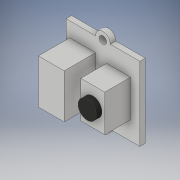
# Autodesk Inventor part: button
Saved by Autodesk Inventor 2019 (Build 230136000, 136)
## iProperties
Created: 2018-06-15
Part Number: button
Material: Generic
Document SubType Name: Modeling
Designer: daniel
Density: 1 g/cm^3
Appearance: Default
Author: daniel
Autodesk Inventor part; units mm, degrees
ref_plane "YZ Plane" through (0, 0, 0) normal (1, 0, 0) x (0, 1, 0)
ref_plane "XZ Plane" through (0, 0, 0) normal (0, 1, 0) x (-1, 0, 0)
ref_plane "XY Plane" through (0, 0, 0) normal (0, 0, 1) x (1, 0, 0)
sketch "Sketch1" plane through (0, 0, 0) normal (0, 0, 1) x (1, 0, 0)
  line L0 (-10, -10) -> (10, -10)
  line L1 (10, -10) -> (10, 10)
  line L2 (10, 10) -> (-10, 10)
  line L3 (-10, 10) -> (-10, -10)
  line L4 (-10, -10) -> (10, 10) construction
  line L5 (10, -10) -> (-10, 10) construction
  arc A0 (2, 10) -> (-2, 10) centre (0, 10) ccw
  arc A1 (-2, -10) -> (2, -10) centre (0, -10) ccw
  point P0 (0, 0)
  dimension "d0" = 20
  dimension "d1" = 20
  dimension "d4" = 4
  dimension "d5" = 4
  constraints: 12 end point, 4 midpoint, 4 point on circle, 4 point on line, 2 centre point, 2 parallel, 1 horizontal, 1 perpendicular
  measures "d0" distance of L2.end L1.end
  measures "d1" distance of L1.end L0.end
  measures "d4" diameter of A0
  measures "d5" diameter of A1
extrude "Extrusion1" add sketch "Sketch1" along normal blind 1.5
sketch "Sketch2" plane through (0, 0, 1.5) normal (0, 0, 1) x (1, 0, 0)
  arc A0 (2, 10) -> (-2, 10) centre (0, 10) ccw projected
  point P0 (0, 0)
  constraints: 1 coincident
hole "Hole1" at (0, 10, 1.5) direction (0, 0, -1) diameter 2 end through all
mirror "Mirror1" about plane through (0, 0, 0) normal (0, 1, 0) of "Hole1"
sketch "Sketch3" plane through (0, 0, 1.5) normal (0, 0, 1) x (1, 0, 0)
  line L0 (1, -5) -> (7.5, -5)
  line L1 (7.5, -5) -> (7.5, 5)
  line L2 (7.5, 5) -> (1, 5)
  line L3 (1, 5) -> (1, -5)
  line L4 (1, -5) -> (7.5, 5) construction
  line L5 (7.5, -5) -> (1, 5) construction
  circle A0 centre (0, 10) radius 1 projected
  line L6 (1, 10) -> (1, 0) construction
  circle A1 centre (0, 10) radius 1 projected
  line L7 (10, -10) -> (10, 10) projected
  line L8 (-14, 0) -> (14, 0) projected
  point P0 (0, 0)
  point P1 (4.25, 0)
  point P2 (4.25, 0)
  dimension "d13" = 2.5
  dimension "d14" = 10
  constraints: 14 end point, 3 midpoint, 2 horizontal alignment, 2 parallel, 2 vertical, 1 collinear, 1 horizontal, 1 perpendicular, 1 point on line, 1 other
  measures "d13" distance between parallel lines of L7 L1
  measures "d14" distance of L0.end L1.end
extrude "Extrusion2" add sketch "Sketch3" along normal blind 7 contours L3 L8 L1 L0 | L3 L2 L1 L8
sketch "Sketch4" plane through (0, 0, 8.5) normal (0, 0, 1) x (1, 0, 0)
  circle A0 centre (4.25, 0) radius 2.5
  line L0 (-14, 0) -> (14, 0) projected
  line L1 (7.5, 5) -> (1, 5) projected
  line L2 (4.25, 5) -> (4.25, 0) construction
  point P0 (0, 0)
  dimension "d17" = 5
  constraints: 2 end point, 1 centre point, 1 midpoint, 1 perpendicular, 1 point on line
  measures "d17" diameter of A0
extrude "Extrusion3" add sketch "Sketch4" along normal blind 1.5
sketch "Sketch5" plane through (0, 0, 1.5) normal (0, 0, 1) x (1, 0, 0)
  line L0 (-9, 6) -> (-2, 6)
  line L1 (-2, 6) -> (-2, -6)
  line L2 (-2, -6) -> (-9, -6)
  line L3 (-9, -6) -> (-9, 6)
  line L4 (-9, 6) -> (-2, -6) construction
  line L5 (-2, 6) -> (-9, -6) construction
  line L6 (-26.8178, 0) -> (16.1363, 0) projected
  line L7 (-10, 10) -> (-10, -10) projected
  point P0 (0, 0)
  point P1 (-5.5, 0)
  point P2 (-5.5, 0)
  dimension "d20" = 7
  dimension "d21" = 12
  dimension "d22" = 1
  constraints: 12 end point, 3 midpoint, 2 parallel, 1 horizontal, 1 perpendicular, 1 point on line
  measures "d20" distance of L1.end L2.end
  measures "d21" distance of L0.end L1.end
  measures "d22" distance between parallel lines of L7 L3
extrude "Extrusion4" add sketch "Sketch5" along normal blind 8.5
body "Solid1"
